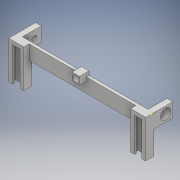
# Autodesk Inventor part: frontAxelHolder 9-1
Saved by Autodesk Inventor 2018 (Build 220112000, 112)
## iProperties
Created: 2019-09-01
Part Number: frontAxelHolder 9-1
Material: Generic
Document SubType Name: Modeling
Designer: Aditya Kendre
Density: 1 g/cm^3
Appearance: Default
Author: Aditya Kendre
Autodesk Inventor part; units mm, degrees
ref_plane "YZ Plane" through (0, 0, 0) normal (1, 0, 0) x (0, 1, 0)
ref_plane "XZ Plane" through (0, 0, 0) normal (0, 1, 0) x (-1, 0, 0)
ref_plane "XY Plane" through (0, 0, 0) normal (0, 0, 1) x (1, 0, 0)
sketch "Sketch1" plane through (0, 0, 0) normal (0, 1, 0) x (-1, 0, 0)
  line L0 (0, 0) -> (145, 0)
  line L1 (145, 0) -> (145, -15)
  line L2 (145, -15) -> (0, -15)
  line L3 (0, -15) -> (0, 0)
  dimension "d0" = 145
  dimension "d1" = 15
  constraints: 8 end point, 2 parallel, 1 horizontal, 1 perpendicular
  measures "d0" distance of L1.end L2.end
  measures "d1" distance of L0.end L1.end
extrude "Extrusion1" add sketch "Sketch1" along normal blind 3
sketch "Sketch2" plane through (0, 3, 0) normal (0, 1, 0) x (1, 0, 0)
  line L0 (-145, 0) -> (0, 0) projected
  line L1 (0, 15) -> (-145, 15) projected
  line L2 (-145, 0) -> (-139, 0)
  line L3 (-139, 0) -> (-139, 15)
  line L4 (-139, 15) -> (-145, 15)
  line L5 (-145, 15) -> (-145, 0)
  line L6 (0, 0) -> (-6, 0)
  line L7 (-6, 0) -> (-6, 15)
  line L8 (-6, 15) -> (0, 15)
  line L9 (0, 15) -> (0, 0)
  dimension "d4" = 6
  dimension "d5" = 6
  constraints: 16 end point, 4 parallel, 2 horizontal, 2 perpendicular, 2 point on line
  measures "d4" distance of L4.end L3.end
  measures "d5" distance of L7.end L8.end
extrude "Extrusion2" add sketch "Sketch2" along normal blind 20 contours L5 L1 L3 L0 | L7 L1 L9 L0
sketch "Sketch3" plane through (0, 0, 0) normal (1, 0, 0) x (0, 0, -1)
  line L0 (0, 3) -> (15, 3) construction
  line L1 (7.5, 3) -> (7.5, 15.5) construction
  circle A0 centre (7.5, 15.5) radius 5
  point P0 (0, 0)
  dimension "d8" = 12.5
  dimension "d9" = 10
  constraints: 2 end point, 1 centre point, 1 coincident, 1 midpoint, 1 vertical
  measures "d8" distance of L1.start L1.end
  measures "d9" diameter of A0
extrude "Extrusion3" cut sketch "Sketch3" against normal blind 156
sketch "Sketch4" plane through (-139, 3, 0) normal (1, 0, 0) x (0, 0, -1)
  circle A0 centre (7.5, 12.5) radius 5 projected
  circle A1 centre (7.5, 12.5) radius 5
  circle A2 centre (7.5, 12.5) radius 5 projected
  circle A3 centre (7.5, 12.5) radius 2.5
  point P0 (0, -3)
  dimension "d12" = 5
  constraints: 2 centre point, 2 coincident
  measures "d12" diameter of A3
extrude "Extrusion4" add sketch "Sketch4" against normal blind 1.5
sketch "Sketch5" plane through (-6, 3, -15) normal (-1, 0, 0) x (0, 0, 1)
  circle A0 centre (7.5, 12.5) radius 2.5 projected
  circle A1 centre (7.5, 12.5) radius 5
  circle A2 centre (7.5, 12.5) radius 2.4999
  point P0 (15, -3)
  constraints: 2 centre point, 2 coincident
extrude "Extrusion5" add sketch "Sketch5" against normal blind 1.5
sketch "Sketch6" plane through (0, 3, 0) normal (0, 1, 0) x (1, 0, 0)
  line L0 (0, 0) -> (-145, 0) projected
  line L1 (-72.5, 0) -> (-76.5, 0)
  line L2 (-76.5, 0) -> (-76.5, -4)
  line L3 (-76.5, -4) -> (-72.5, -4)
  line L4 (-72.5, -4) -> (-72.5, 0)
  line L5 (-72.5, 0) -> (-68.5, 0)
  line L6 (-68.5, 0) -> (-68.5, -4)
  line L7 (-68.5, -4) -> (-72.5, -4)
  line L8 (-72.5, -4) -> (-72.5, 0)
  dimension "d17" = 4
  dimension "d18" = 4
  dimension "d19" = 4
  constraints: 16 end point, 4 parallel, 2 horizontal, 2 perpendicular, 1 midpoint, 1 point on line
  measures "d17" distance of L3.end L2.end
  measures "d18" distance of L2.end L1.end
  measures "d19" distance of L6.end L7.end
extrude "Extrusion6" add sketch "Sketch6" against normal blind 3
sketch "Sketch7" plane through (0, 3, 0) normal (0, 1, 0) x (1, 0, 0)
  circle A0 centre (-72.5, 0) radius 3.2
  line L0 (-68.5, 0) -> (-68.5, -4) projected
  line L1 (-68.5, -4) -> (-76.5, -4)
  line L2 (-76.5, -4) -> (-76.5, 4)
  line L3 (-76.5, 4) -> (-68.5, 4)
  line L4 (-68.5, 4) -> (-68.5, -4)
  point P0 (0, 0)
  dimension "d22" = 6.4
  dimension "d23" = 8
  constraints: 8 end point, 2 parallel, 1 centre point, 1 horizontal, 1 perpendicular
  measures "d22" diameter of A0
  measures "d23" distance of L1.end L2.end
extrude "Extrusion7" add sketch "Sketch7" against normal blind 10
sketch "Sketch8" plane through (-72.5, 0, 0) normal (0, -1, 0) x (1, 0, 0)
  point P0 (72.5, 0)
sketch "Sketch9" plane through (-72.5, 0, 0) normal (0, -1, 0) x (1, 0, 0)
  circle A0 centre (0, 0) radius 3.2
  point P0 (72.5, 0)
  constraints: 1 centre point
extrude "Extrusion8" cut sketch "Sketch9" against normal blind 7.5
sketch "Sketch10" plane through (0, 0, 0) normal (0, -1, 0) x (1, 0, 0)
  line L0 (0, 0) -> (0, -15) construction
  line L1 (0, 0) -> (-16, 0) construction
  line L2 (-16, 0) -> (-16, -25) construction
  line L3 (-16, -25) -> (0, -25) construction
  line L4 (0, -25) -> (0, 0) construction
  line L5 (-145, -15) -> (-145, 0) construction
  line L6 (-145, 0) -> (-129, 0) construction
  line L7 (-129, 0) -> (-129, -25) construction
  line L8 (-129, -25) -> (-145, -25) construction
  line L9 (-145, -25) -> (-145, 0) construction
  line L10 (0, -25) -> (-2, -25)
  line L11 (-2, -25) -> (-2, -2)
  line L12 (-2, -2) -> (-14, -2)
  line L13 (-14, -2) -> (-14, -25)
  line L14 (-16, -25) -> (-16, 0)
  line L15 (-68.5, 0) -> (-6, 0) projected
  line L16 (-6, 0) -> (0, 0) projected
  line L17 (0, 0) -> (-16, 0)
  line L18 (0, -25) -> (0, 0)
  line L19 (0, -2.5) -> (-4.5, -2.5) projected
  line L20 (-129, -25) -> (-129, 0)
  line L21 (-145, 0) -> (-139, 0) projected
  line L22 (-145, 0) -> (-145, -25)
  line L23 (-145, -25) -> (-143, -25)
  line L24 (-143, -25) -> (-143, -2)
  line L25 (-143, -2) -> (-131, -2)
  line L26 (-131, -2) -> (-131, -25)
  line L27 (-129, -25) -> (-131, -25)
  line L28 (-14, -25) -> (-16, -25)
  line L29 (-129, 0) -> (-145, 0)
  dimension "d28" = 16
  dimension "d29" = 25
  dimension "d30" = 16
  dimension "d31" = 25
  dimension "d32" = 2
  dimension "d33" = 23
  dimension "d34" = 12
  dimension "d35" = 2
  dimension "d36" = 23
  dimension "d37" = 12
  constraints: 48 end point, 12 perpendicular, 4 parallel, 4 point on line, 3 horizontal, 2 collinear, 1 vertical
  measures "d28" distance of L3.end L2.end
  measures "d29" distance of L2.end L1.end
  measures "d30" distance of L7.end L8.end
  measures "d31" distance of L6.end L7.end
  measures "d32" distance of L3.end L10.end
  measures "d33" distance of L10.end L11.end
  measures "d34" distance of L11.end L12.end
  measures "d35" distance of L8.end L23.end
  measures "d36" distance of L23.end L24.end
  measures "d37" distance of L24.end L25.end
extrude "Extrusion9" add sketch "Sketch10" along normal blind 3.5
sketch "Sketch11" plane through (0, 0, 0) normal (0, 1, 0) x (1, 0, 0)
  line L0 (0, 25) -> (0, 0) projected
  line L1 (-16, 0) -> (-16, 25) projected
  line L2 (0, 25) -> (-16, 25)
  line L3 (-16, 25) -> (-16, 15.0002)
  line L4 (-16, 15.0002) -> (0, 15.0002)
  line L5 (0, 15.0002) -> (0, 25)
  line L6 (-131, 25) -> (-129, 25) projected
  line L7 (-145, 0) -> (-145, 25) projected
  line L8 (-129, 25) -> (-145, 25)
  line L9 (-145, 25) -> (-145, 15.0002)
  line L10 (-145, 15.0002) -> (-129, 15.0002)
  line L11 (-129, 15.0002) -> (-129, 25)
  constraints: 16 end point, 4 parallel, 3 point on line, 2 horizontal, 2 perpendicular
extrude "Extrusion10" add sketch "Sketch11" along normal blind 3
sketch "Sketch12" plane through (0, -3.5, 0) normal (0, -1, 0) x (1, 0, 0)
  line L0 (0, -25) -> (0, 0) projected
  line L1 (0, 0) -> (-16, 0) projected
  line L2 (0, -25) -> (-4, -25)
  line L3 (-4, -25) -> (-4, 0)
  line L4 (-4, 0) -> (0, 0)
  line L5 (0, 0) -> (0, -25)
  line L6 (-16, 0) -> (-16, -25) projected
  line L7 (0, 0) -> (-16, 0)
  line L8 (-16, 0) -> (-16, -4)
  line L9 (-16, -4) -> (0, -4)
  line L10 (0, -4) -> (0, 0)
  line L11 (-16, -25) -> (-12, -25)
  line L12 (-12, -25) -> (-12, 0)
  line L13 (-12, 0) -> (-16, 0)
  line L14 (-16, 0) -> (-16, -25)
  line L15 (-129, 0) -> (-145, 0) projected
  line L16 (-129, -25) -> (-133, -25)
  line L17 (-133, -25) -> (-133, 0)
  line L18 (-133, 0) -> (-129, 0)
  line L19 (-129, 0) -> (-129, -25)
  line L20 (-145, -25) -> (-143, -25) projected
  line L21 (-145, -25) -> (-141, -25)
  line L22 (-141, -25) -> (-141, 0)
  line L23 (-141, 0) -> (-145, 0)
  line L24 (-145, 0) -> (-145, -25)
  line L25 (-129, 0) -> (-145, 0)
  line L26 (-145, 0) -> (-145, -4)
  line L27 (-145, -4) -> (-129, -4)
  line L28 (-129, -4) -> (-129, 0)
  dimension "d42" = 4
  dimension "d43" = 4
  dimension "d44" = 4
  dimension "d45" = 4
  dimension "d46" = 4
  constraints: 48 end point, 12 parallel, 6 horizontal, 6 perpendicular, 6 point on line
  measures "d42" distance of L3.end L4.end
  measures "d43" distance of L8.end L7.end
  measures "d44" distance of L13.end L12.end
  measures "d45" distance of L17.end L18.end
  measures "d46" distance of L23.end L22.end
extrude "Extrusion11" add sketch "Sketch12" along normal blind 2
sketch "Sketch13" plane through (-2, 0, -25) normal (0, 0, -1) x (-1, 0, 0)
  line L0 (-2, 3) -> (14, 3) projected
  line L1 (2, -5.5) -> (-2, -5.5) projected
  line L2 (-2, 3) -> (0, 3)
  line L3 (0, 3) -> (0, -5.5)
  line L4 (0, -5.5) -> (-2, -5.5)
  line L5 (-2, -5.5) -> (-2, 3)
  line L6 (0, 0) -> (0, -3.5) projected
  line L7 (2, -5.5) -> (0, -5.5)
  line L8 (0, -5.5) -> (0, -3.5)
  line L9 (0, -3.5) -> (2, -3.5)
  line L10 (2, -3.5) -> (2, -5.5)
  line L11 (14, -5.5) -> (10, -5.5) projected
  line L12 (10, -3.5) -> (14, -3.5)
  line L13 (14, -3.5) -> (14, -5.5)
  line L14 (14, -5.5) -> (10, -5.5)
  line L15 (10, -5.5) -> (10, -3.5)
  line L16 (66.5, 3) -> (4, 3) projected
  line L17 (14, -3.5) -> (12, -3.5)
  line L18 (12, -3.5) -> (12, 3)
  line L19 (12, 3) -> (14, 3)
  line L20 (14, 3) -> (14, -3.5)
  line L21 (0, 0) -> (12, 0) projected
  line L22 (12, 3) -> (0, 3)
  line L23 (0, 3) -> (0, 0)
  line L24 (0, 0) -> (12, 0)
  line L25 (12, 0) -> (12, 3)
  line L26 (127, 0) -> (127, 3) projected
  line L27 (143, 3) -> (143, -5.5) projected
  line L28 (127, 3) -> (143, 3)
  line L29 (143, 3) -> (143, 0)
  line L30 (143, 0) -> (127, 0)
  line L31 (127, 0) -> (127, 3)
  line L32 (143, -5.5) -> (139, -5.5) projected
  line L33 (143, 0) -> (141, 0)
  line L34 (141, 0) -> (141, -5.5)
  line L35 (141, -5.5) -> (143, -5.5)
  line L36 (143, -5.5) -> (143, 0)
  line L37 (141, -3.5) -> (139, -3.5) projected
  line L38 (139, -3.5) -> (141, -3.5)
  line L39 (141, -3.5) -> (141, -5.5)
  line L40 (141, -5.5) -> (139, -5.5)
  line L41 (139, -5.5) -> (139, -3.5)
  line L42 (127, 0) -> (14, 0) projected
  line L43 (131, -5.5) -> (127, -5.5) projected
  line L44 (127, 0) -> (129, 0)
  line L45 (129, 0) -> (129, -5.5)
  line L46 (129, -5.5) -> (127, -5.5)
  line L47 (127, -5.5) -> (127, 0)
  line L48 (131, -3.5) -> (131, -5.5) projected
  line L49 (131, -3.5) -> (129, -3.5)
  line L50 (129, -3.5) -> (129, -5.5)
  line L51 (129, -5.5) -> (131, -5.5)
  line L52 (131, -5.5) -> (131, -3.5)
  point P0 (-2, 0)
  constraints: 80 end point, 20 parallel, 10 horizontal, 10 perpendicular, 3 midpoint, 3 point on line
extrude "Extrusion12" add sketch "Sketch13" along normal blind 15 and the other way blind 16.5
sketch "Sketch14" plane through (-145, 3, -15) normal (-1, 0, 0) x (0, 0, 1)
  circle A0 centre (7.5, 12.5) radius 2.5 projected
  circle A1 centre (7.5, 12.5) radius 5.5
  point P0 (15, -3)
  dimension "d53" = 11
  constraints: 1 centre point, 1 coincident
  measures "d53" diameter of A1
extrude "Extrusion13" cut sketch "Sketch14" against normal blind 4.5
sketch "Sketch15" plane through (0, 3, -15) normal (1, 0, 0) x (0, 0, -1)
  circle A0 centre (-7.5, 12.5) radius 5.5 projected
  circle A1 centre (-7.5, 12.5) radius 5.5
  point P0 (-15, -3)
  constraints: 1 centre point, 1 coincident
extrude "Extrusion14" cut sketch "Sketch15" against normal blind 4.5
body "Solid1"
